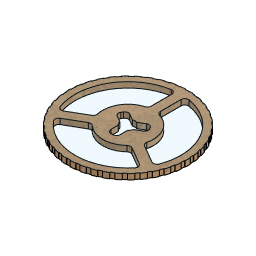
wheel + hub hole v3 (Autodesk Fusion 360 design; units mm, degrees)
Autodesk Fusion 360 part; units mm, degrees
note: some values were not read from the file. Chosen so that the rebuilt part matches the saved one: which bodies a step acts on.
sketch "Sketch1" plane through (0, 0, 0) normal (0, 0, 1) x (1, 0, 0)
  line L0 (-14.6554, 9.616) -> (-15.6554, 7.884)
  arc A0 (14.6554, 9.616) -> (9.1913, 11.0801) centre (11.1913, 7.616) ccw
  line L1 (-1, -17.5) -> (1, -17.5)
  arc A1 (2.3412, 7.1252) -> (-2.3412, 7.1252) centre (0, 0) ccw
  line L2 (15.6554, 7.884) -> (14.6554, 9.616)
  arc A2 (1, -17.5) -> (5, -13.5) centre (1, -13.5) ccw
  arc A3 (-5, -13.5) -> (-1, -17.5) centre (-1, -13.5) ccw
  arc A4 (-15.6554, 7.884) -> (-14.1913, 2.4199) centre (-12.1913, 5.884) ccw
  arc A5 (5, -5.5902) -> (7.3412, -1.535) centre (0, 0) ccw
  arc A6 (14.1913, 2.4199) -> (15.6554, 7.884) centre (12.1913, 5.884) ccw
  line L3 (-14.1913, 2.4199) -> (-7.3412, -1.535)
  arc A7 (-9.1913, 11.0801) -> (-14.6554, 9.616) centre (-11.1913, 7.616) ccw
  line L4 (-5, -5.5902) -> (-5, -13.5)
  line L5 (7.3412, -1.535) -> (14.1913, 2.4199)
  arc A8 (-7.3412, -1.535) -> (-5, -5.5902) centre (0, 0) ccw
  line L6 (-2.3412, 7.1252) -> (-9.1913, 11.0801)
  line L7 (5, -13.5) -> (5, -5.5902)
  line L8 (9.1913, 11.0801) -> (2.3412, 7.1252)
  circle A9 centre (0, 0) radius 65
  dimension "d1" = 130
  constraint concentric A1 A9
  measures "d1" diameter of A9
extrude "Extrude1" add sketch "Sketch1" against normal blind 6 makes body 1
sketch "Sketch2" plane through (0, 0, 0) normal (0, 0, 1) x (-1, 0, 0)
  line L0 (-2.3412, -7.1252) -> (-9.1913, -11.0801)
  arc A0 (-14.6554, -9.616) -> (-9.1913, -11.0801) centre (-11.1913, -7.616) ccw
  line L1 (-14.6554, -9.616) -> (-15.6554, -7.884)
  arc A1 (-14.1913, -2.4199) -> (-15.6554, -7.884) centre (-12.1913, -5.884) ccw
  line L2 (-14.1913, -2.4199) -> (-7.3412, 1.535)
  arc A2 (-5, 5.5902) -> (-7.3412, 1.535) centre (0, 0) ccw
  line L3 (-5, 5.5902) -> (-5, 13.5)
  arc A3 (-1, 17.5) -> (-5, 13.5) centre (-1, 13.5) ccw
  line L4 (-1, 17.5) -> (1, 17.5)
  arc A4 (5, 13.5) -> (1, 17.5) centre (1, 13.5) ccw
  line L5 (5, 13.5) -> (5, 5.5902)
  arc A5 (7.3412, 1.535) -> (5, 5.5902) centre (0, 0) ccw
  line L6 (7.3412, 1.535) -> (14.1913, -2.4199)
  arc A6 (15.6554, -7.884) -> (14.1913, -2.4199) centre (12.1913, -5.884) ccw
  line L7 (15.6554, -7.884) -> (14.6554, -9.616)
  arc A7 (9.1913, -11.0801) -> (14.6554, -9.616) centre (11.1913, -7.616) ccw
  line L8 (9.1913, -11.0801) -> (2.3412, -7.1252)
  arc A8 (-2.3412, -7.1252) -> (2.3412, -7.1252) centre (0, 0) ccw
  circle A9 centre (0, 0) radius 65
  circle A10 centre (0, 0) radius 27.5
  circle A11 centre (0, 0) radius 57.5
  dimension "d4" = 55
  dimension "d5" = 115
  constraint concentric A2 A10
  constraint concentric A2 A11
  measures "d4" diameter of A10
  measures "d5" diameter of A11
extrude "Extrude2" cut sketch "Sketch2" against normal blind 6 contours A11 bodies 1 makes body 2 at (62.0439, -6.0859, 0)
sketch "Sketch3" plane through (0, 0, 0) normal (0, 0, 1) x (-1, 0, 0)
  circle A0 centre (0, 0) radius 27.5
  line L0 (-2.3412, -7.1252) -> (-9.1913, -11.0801)
  arc A1 (-14.6554, -9.616) -> (-9.1913, -11.0801) centre (-11.1913, -7.616) ccw
  line L1 (-14.6554, -9.616) -> (-15.6554, -7.884)
  arc A2 (-14.1913, -2.4199) -> (-15.6554, -7.884) centre (-12.1913, -5.884) ccw
  line L2 (-14.1913, -2.4199) -> (-7.3412, 1.535)
  arc A3 (-5, 5.5902) -> (-7.3412, 1.535) centre (0, 0) ccw
  line L3 (-5, 5.5902) -> (-5, 13.5)
  arc A4 (-1, 17.5) -> (-5, 13.5) centre (-1, 13.5) ccw
  line L4 (-1, 17.5) -> (1, 17.5)
  arc A5 (5, 13.5) -> (1, 17.5) centre (1, 13.5) ccw
  line L5 (5, 13.5) -> (5, 5.5902)
  arc A6 (7.3412, 1.535) -> (5, 5.5902) centre (0, 0) ccw
  line L6 (7.3412, 1.535) -> (14.1913, -2.4199)
  arc A7 (15.6554, -7.884) -> (14.1913, -2.4199) centre (12.1913, -5.884) ccw
  line L7 (15.6554, -7.884) -> (14.6554, -9.616)
  arc A8 (9.1913, -11.0801) -> (14.6554, -9.616) centre (11.1913, -7.616) ccw
  line L8 (9.1913, -11.0801) -> (2.3412, -7.1252)
  arc A9 (-2.3412, -7.1252) -> (2.3412, -7.1252) centre (0, 0) ccw
  line L9 (0, -27.5) -> (0, -58) construction
  line L10 (0, -58) -> (-5, -58) construction
  line L11 (-5, -58) -> (-5, -26) construction
  line L12 (-5, -26) -> (5, -26) construction
  line L13 (5, -26) -> (5, -58) construction
  line L14 (0, -58) -> (5, -58) construction
  line L15 (5, -27.0416) -> (5, -58)
  line L16 (5, -58) -> (-5, -58)
  line L17 (-5, -58) -> (-5, -26)
  line L18 (-5, -26) -> (5, -26)
  line L19 (5, -27.0416) -> (5, -26)
  line L20 (25.0167, 8.6699) -> (20.0167, 17.3301)
  line L21 (20.9187, 17.8509) -> (20.0167, 17.3301)
  line L22 (20.9187, 17.8509) -> (47.7295, 33.3301)
  line L23 (52.7295, 24.6699) -> (25.0167, 8.6699) construction
  line L24 (47.7295, 33.3301) -> (52.7295, 24.6699)
  line L25 (-20.0167, 17.3301) -> (-25.0167, 8.6699)
  line L26 (-25.9187, 9.1907) -> (-25.0167, 8.6699)
  line L27 (-25.9187, 9.1907) -> (-52.7295, 24.6699)
  line L28 (-47.7295, 33.3301) -> (-20.0167, 17.3301) construction
  line L29 (-52.7295, 24.6699) -> (-47.7295, 33.3301)
  line L30 (-20.0167, 17.3301) -> (-47.7295, 33.3301)
  line L31 (25.0167, 8.6699) -> (52.7295, 24.6699)
  dimension "d9" = 360
  constraint coincident A0 L9.start
  constraint vertical L9
  constraint perpendicular L9 L10
  constraint perpendicular L10 L11
  constraint perpendicular L11 L12
  constraint perpendicular L12 L13
  constraint perpendicular L13 L14
  constraint coincident L13 L15.start
  constraint coincident A0 L15.start
  constraint perpendicular L11 L16
  constraint perpendicular L12 L19
extrude "Extrude3" add sketch "Sketch3" against normal blind 6 contours A0 L15 L16 L17 | A0 L22 L24 L31 | A0 L27 L29 L30 bodies 1 2
fillet "Fillet1" radius 4 12 edges at (-20.9187, -17.8509, -3) (-25.9187, -9.1907, -3) (-47.1078, -32.9712, -3) (-52.1078, -24.311, -3) (20.9187, -17.8509, -3) (25.9187, -9.1907, -3) (47.1078, -32.9712, -3) (52.1078, -24.311, -3) (5, 57.2822, -3) (-5, 57.2822, -3) (5, 27.0416, -3) (-5, 27.0416, -3) on bodies 1
sketch "Sketch4" plane through (0, 0, -6) normal (0, 0, -1) x (1, 0, 0)
  arc A0 (9.6729, -56.6806) -> (53.9232, 19.9633) centre (0, 0) ccw
  arc A1 (5, -52.7376) -> (9.6729, -56.6806) centre (9, -52.7376) ccw
  line L0 (5, -52.7376) -> (5, -30.1869)
  arc A2 (7.8571, -26.3537) -> (5, -30.1869) centre (9, -30.1869) ccw
  arc A3 (7.8571, -26.3537) -> (26.7515, 6.3723) centre (0, 0) ccw
  arc A4 (28.6426, 10.7633) -> (26.7515, 6.3723) centre (30.6426, 7.2992) ccw
  line L1 (28.6426, 10.7633) -> (48.1721, 22.0387)
  arc A5 (53.9232, 19.9633) -> (48.1721, 22.0387) centre (50.1721, 18.5746) ccw
  line L2 (43.1721, 30.6989) -> (23.6426, 19.4236)
  arc A6 (18.8944, 19.9813) -> (23.6426, 19.4236) centre (21.6426, 22.8877) ccw
  arc A7 (18.8944, 19.9813) -> (-18.8944, 19.9813) centre (0, 0) ccw
  arc A8 (-23.6426, 19.4236) -> (-18.8944, 19.9813) centre (-21.6426, 22.8877) ccw
  line L3 (-23.6426, 19.4236) -> (-43.1721, 30.6989)
  arc A9 (-44.2503, 36.7173) -> (-43.1721, 30.6989) centre (-41.1721, 34.163) ccw
  arc A10 (44.2503, 36.7173) -> (-44.2503, 36.7173) centre (0, 0) ccw
  arc A11 (43.1721, 30.6989) -> (44.2503, 36.7173) centre (41.1721, 34.163) ccw
  line L4 (-5, -30.1869) -> (-5, -52.7376)
  arc A12 (-9.6729, -56.6806) -> (-5, -52.7376) centre (-9, -52.7376) ccw
  arc A13 (-53.9232, 19.9633) -> (-9.6729, -56.6806) centre (0, 0) ccw
  arc A14 (-48.1721, 22.0387) -> (-53.9232, 19.9633) centre (-50.1721, 18.5746) ccw
  line L5 (-48.1721, 22.0387) -> (-28.6426, 10.7633)
  arc A15 (-26.7515, 6.3723) -> (-28.6426, 10.7633) centre (-30.6426, 7.2992) ccw
  arc A16 (-26.7515, 6.3723) -> (-7.8571, -26.3537) centre (0, 0) ccw
  arc A17 (-5, -30.1869) -> (-7.8571, -26.3537) centre (-9, -30.1869) ccw
  circle A18 centre (0, 0) radius 65
  line L6 (9.1913, -11.0801) -> (2.3412, -7.1252)
  arc A19 (-2.3412, -7.1252) -> (2.3412, -7.1252) centre (0, 0) ccw
  line L7 (-2.3412, -7.1252) -> (-9.1913, -11.0801)
  arc A20 (-14.6554, -9.616) -> (-9.1913, -11.0801) centre (-11.1913, -7.616) ccw
  line L8 (-14.6554, -9.616) -> (-15.6554, -7.884)
  arc A21 (-14.1913, -2.4199) -> (-15.6554, -7.884) centre (-12.1913, -5.884) ccw
  line L9 (-14.1913, -2.4199) -> (-7.3412, 1.535)
  arc A22 (-5, 5.5902) -> (-7.3412, 1.535) centre (0, 0) ccw
  line L10 (-5, 5.5902) -> (-5, 13.5)
  arc A23 (-1, 17.5) -> (-5, 13.5) centre (-1, 13.5) ccw
  line L11 (-1, 17.5) -> (1, 17.5)
  arc A24 (5, 13.5) -> (1, 17.5) centre (1, 13.5) ccw
  line L12 (5, 13.5) -> (5, 5.5902)
  arc A25 (7.3412, 1.535) -> (5, 5.5902) centre (0, 0) ccw
  line L13 (7.3412, 1.535) -> (14.1913, -2.4199)
  arc A26 (15.6554, -7.884) -> (14.1913, -2.4199) centre (12.1913, -5.884) ccw
  line L14 (15.6554, -7.884) -> (14.6554, -9.616)
  arc A27 (9.1913, -11.0801) -> (14.6554, -9.616) centre (11.1913, -7.616) ccw
  line L15 (2, -65.5) -> (-2, -65.5) construction
  line L16 (-2, -65.5) -> (-2, -64.5) construction
  line L17 (-2, -64.5) -> (2, -64.5) construction
  line L18 (2, -64.5) -> (2, -65.5) construction
  line L19 (2, -65.5) -> (-2, -64.5) construction
  line L20 (-2, -65.5) -> (2, -64.5) construction
  line L21 (-2, -64.5) -> (2, -64.5) construction
  line L22 (2, -64.5) -> (2, -65.5) construction
  line L23 (2, -65.5) -> (-2, -65.5) construction
  line L24 (-2, -65.5) -> (-2, -64.5) construction
  line L25 (-2, -64.5) -> (2, -64.5)
  line L26 (2, -64.5) -> (2, -65.5)
  line L27 (2, -65.5) -> (-2, -65.5)
  line L28 (-2, -65.5) -> (-2, -64.5)
  point P0 (0, -65)
  dimension "d14" = 1
  constraint horizontal L15
  constraint perpendicular L15 L16
  constraint parallel L15 L17
  constraint parallel L16 L18
  constraint coincident L19 P0
  constraint coincident L20 P0
  constraint coincident A18 P0
  constraint horizontal L21
  constraint vertical L22
  constraint horizontal L23
  constraint vertical L24
  constraint horizontal L25
  constraint vertical L26
  constraint horizontal L27
  constraint vertical L28
  measures "d14" distance of L15.end L16.end
extrude "Extrude4" cut sketch "Sketch4" against normal blind 6 contours A18 L25 L26 L28 picked at (-0.2223, -64.6655) bodies 1
pattern_circular "C-Pattern1" count 42 over 360 about axis through (0, 0, 1.75) along (0, 0, 1) of "Extrude4"
sketch "Sketch5" plane through (0, 0, 0) normal (0, 0, 1) x (-1, 0, 0)
  line L0 (-11.6608, -63.9455) -> (-11.5909, -63.4815)
  line L1 (-11.5909, -63.4815) -> (-7.6356, -64.0777)
  line L2 (-7.6356, -64.0777) -> (-7.7055, -64.5417)
  arc A0 (-7.7055, -64.5417) -> (-2, -64.9692) centre (0, 0) ccw
  line L3 (-2, -64.9692) -> (-2, -64.5)
  line L4 (-2, -64.5) -> (2, -64.5)
  line L5 (2, -64.5) -> (2, -64.9692)
  arc A1 (2, -64.9692) -> (7.7055, -64.5417) centre (0, 0) ccw
  line L6 (7.7055, -64.5417) -> (7.6356, -64.0777)
  line L7 (7.6356, -64.0777) -> (11.5909, -63.4815)
  line L8 (11.5909, -63.4815) -> (11.6608, -63.9455)
  arc A2 (11.6608, -63.9455) -> (17.2389, -62.6723) centre (0, 0) ccw
  line L9 (17.2389, -62.6723) -> (17.1006, -62.224)
  line L10 (17.1006, -62.224) -> (20.9229, -61.0449)
  line L11 (20.9229, -61.0449) -> (21.0612, -61.4933)
  arc A3 (21.0612, -61.4933) -> (26.3872, -59.403) centre (0, 0) ccw
  line L12 (26.3872, -59.403) -> (26.1836, -58.9803)
  line L13 (26.1836, -58.9803) -> (29.7874, -57.2447)
  line L14 (29.7874, -57.2447) -> (29.991, -57.6675)
  arc A4 (29.991, -57.6675) -> (34.946, -54.8067) centre (0, 0) ccw
  line L15 (34.946, -54.8067) -> (34.6817, -54.419)
  line L16 (34.6817, -54.419) -> (37.9866, -52.1658)
  line L17 (37.9866, -52.1658) -> (38.2509, -52.5535)
  arc A5 (38.2509, -52.5535) -> (42.7242, -48.9862) centre (0, 0) ccw
  line L18 (42.7242, -48.9862) -> (42.405, -48.6422)
  line L19 (42.405, -48.6422) -> (45.3372, -45.9215)
  line L20 (45.3372, -45.9215) -> (45.6564, -46.2655)
  arc A6 (45.6564, -46.2655) -> (49.548, -42.0713) centre (0, 0) ccw
  line L21 (49.548, -42.0713) -> (49.1812, -41.7788)
  line L22 (49.1812, -41.7788) -> (51.6751, -38.6514)
  line L23 (51.6751, -38.6514) -> (52.042, -38.944)
  arc A7 (52.042, -38.944) -> (55.265, -34.2167) centre (0, 0) ccw
  line L24 (55.265, -34.2167) -> (54.8586, -33.9821)
  line L25 (54.8586, -33.9821) -> (56.8586, -30.5179)
  line L26 (56.8586, -30.5179) -> (57.265, -30.7526)
  arc A8 (57.265, -30.7526) -> (59.7475, -25.5977) centre (0, 0) ccw
  line L27 (59.7475, -25.5977) -> (59.3107, -25.4262)
  line L28 (59.3107, -25.4262) -> (60.772, -21.7027)
  line L29 (60.772, -21.7027) -> (61.2088, -21.8742)
  arc A9 (61.2088, -21.8742) -> (62.8953, -16.4069) centre (0, 0) ccw
  line L30 (62.8953, -16.4069) -> (62.4378, -16.3025)
  line L31 (62.4378, -16.3025) -> (63.3279, -12.4027)
  line L32 (63.3279, -12.4027) -> (63.7854, -12.5072)
  arc A10 (63.7854, -12.5072) -> (64.6381, -6.8496) centre (0, 0) ccw
  line L33 (64.6381, -6.8496) -> (64.1702, -6.8145)
  line L34 (64.1702, -6.8145) -> (64.4691, -2.8257)
  line L35 (64.4691, -2.8257) -> (64.937, -2.8607)
  arc A11 (64.937, -2.8607) -> (64.937, 2.8607) centre (0, 0) ccw
  line L36 (64.937, 2.8607) -> (64.4691, 2.8257)
  line L37 (64.4691, 2.8257) -> (64.1702, 6.8145)
  line L38 (64.1702, 6.8145) -> (64.6381, 6.8496)
  arc A12 (64.6381, 6.8496) -> (63.7854, 12.5072) centre (0, 0) ccw
  line L39 (63.7854, 12.5072) -> (63.3279, 12.4027)
  line L40 (63.3279, 12.4027) -> (62.4378, 16.3025)
  line L41 (62.4378, 16.3025) -> (62.8953, 16.4069)
  arc A13 (62.8953, 16.4069) -> (61.2088, 21.8742) centre (0, 0) ccw
  line L42 (61.2088, 21.8742) -> (60.772, 21.7027)
  line L43 (60.772, 21.7027) -> (59.3107, 25.4262)
  line L44 (59.3107, 25.4262) -> (59.7475, 25.5977)
  arc A14 (59.7475, 25.5977) -> (57.265, 30.7526) centre (0, 0) ccw
  line L45 (57.265, 30.7526) -> (56.8586, 30.5179)
  line L46 (56.8586, 30.5179) -> (54.8586, 33.9821)
  line L47 (54.8586, 33.9821) -> (55.265, 34.2167)
  arc A15 (55.265, 34.2167) -> (52.042, 38.944) centre (0, 0) ccw
  line L48 (52.042, 38.944) -> (51.6751, 38.6514)
  line L49 (51.6751, 38.6514) -> (49.1812, 41.7788)
  line L50 (49.1812, 41.7788) -> (49.548, 42.0713)
  arc A16 (49.548, 42.0713) -> (45.6564, 46.2655) centre (0, 0) ccw
  line L51 (45.6564, 46.2655) -> (45.3372, 45.9215)
  line L52 (45.3372, 45.9215) -> (42.405, 48.6422)
  line L53 (42.405, 48.6422) -> (42.7242, 48.9862)
  arc A17 (42.7242, 48.9862) -> (38.2509, 52.5535) centre (0, 0) ccw
  line L54 (38.2509, 52.5535) -> (37.9866, 52.1658)
  line L55 (37.9866, 52.1658) -> (34.6817, 54.419)
  line L56 (34.6817, 54.419) -> (34.946, 54.8067)
  arc A18 (34.946, 54.8067) -> (29.991, 57.6675) centre (0, 0) ccw
  line L57 (29.991, 57.6675) -> (29.7874, 57.2447)
  line L58 (29.7874, 57.2447) -> (26.1836, 58.9803)
  line L59 (26.1836, 58.9803) -> (26.3872, 59.403)
  arc A19 (26.3872, 59.403) -> (21.0612, 61.4933) centre (0, 0) ccw
  line L60 (21.0612, 61.4933) -> (20.9229, 61.0449)
  line L61 (20.9229, 61.0449) -> (17.1006, 62.224)
  line L62 (17.1006, 62.224) -> (17.2389, 62.6723)
  arc A20 (17.2389, 62.6723) -> (11.6608, 63.9455) centre (0, 0) ccw
  line L63 (11.6608, 63.9455) -> (11.5909, 63.4815)
  line L64 (11.5909, 63.4815) -> (7.6356, 64.0777)
  line L65 (7.6356, 64.0777) -> (7.7055, 64.5417)
  arc A21 (7.7055, 64.5417) -> (2, 64.9692) centre (0, 0) ccw
  line L66 (2, 64.9692) -> (2, 64.5)
  line L67 (2, 64.5) -> (-2, 64.5)
  line L68 (-2, 64.5) -> (-2, 64.9692)
  arc A22 (-2, 64.9692) -> (-7.7055, 64.5417) centre (0, 0) ccw
  line L69 (-7.7055, 64.5417) -> (-7.6356, 64.0777)
  line L70 (-7.6356, 64.0777) -> (-11.5909, 63.4815)
  line L71 (-11.5909, 63.4815) -> (-11.6608, 63.9455)
  arc A23 (-11.6608, 63.9455) -> (-17.2389, 62.6723) centre (0, 0) ccw
  line L72 (-17.2389, 62.6723) -> (-17.1006, 62.224)
  line L73 (-17.1006, 62.224) -> (-20.9229, 61.0449)
  line L74 (-20.9229, 61.0449) -> (-21.0612, 61.4933)
  arc A24 (-21.0612, 61.4933) -> (-26.3872, 59.403) centre (0, 0) ccw
  line L75 (-26.3872, 59.403) -> (-26.1836, 58.9803)
  line L76 (-26.1836, 58.9803) -> (-29.7874, 57.2447)
  line L77 (-29.7874, 57.2447) -> (-29.991, 57.6675)
  arc A25 (-29.991, 57.6675) -> (-34.946, 54.8067) centre (0, 0) ccw
  line L78 (-34.946, 54.8067) -> (-34.6817, 54.419)
  line L79 (-34.6817, 54.419) -> (-37.9866, 52.1658)
  line L80 (-37.9866, 52.1658) -> (-38.2509, 52.5535)
  arc A26 (-38.2509, 52.5535) -> (-42.7242, 48.9862) centre (0, 0) ccw
  line L81 (-42.7242, 48.9862) -> (-42.405, 48.6422)
  line L82 (-42.405, 48.6422) -> (-45.3372, 45.9215)
  line L83 (-45.3372, 45.9215) -> (-45.6564, 46.2655)
  arc A27 (-45.6564, 46.2655) -> (-49.548, 42.0713) centre (0, 0) ccw
  line L84 (-49.548, 42.0713) -> (-49.1812, 41.7788)
  line L85 (-49.1812, 41.7788) -> (-51.6751, 38.6514)
  line L86 (-51.6751, 38.6514) -> (-52.042, 38.944)
  arc A28 (-52.042, 38.944) -> (-55.265, 34.2167) centre (0, 0) ccw
  line L87 (-55.265, 34.2167) -> (-54.8586, 33.9821)
  line L88 (-54.8586, 33.9821) -> (-56.8586, 30.5179)
  line L89 (-56.8586, 30.5179) -> (-57.265, 30.7526)
  arc A29 (-57.265, 30.7526) -> (-59.7475, 25.5977) centre (0, 0) ccw
  line L90 (-59.7475, 25.5977) -> (-59.3107, 25.4262)
  line L91 (-59.3107, 25.4262) -> (-60.772, 21.7027)
  line L92 (-60.772, 21.7027) -> (-61.2088, 21.8742)
  arc A30 (-61.2088, 21.8742) -> (-62.8953, 16.4069) centre (0, 0) ccw
  line L93 (-62.8953, 16.4069) -> (-62.4378, 16.3025)
  line L94 (-62.4378, 16.3025) -> (-63.3279, 12.4027)
  line L95 (-63.3279, 12.4027) -> (-63.7854, 12.5072)
  arc A31 (-63.7854, 12.5072) -> (-64.6381, 6.8496) centre (0, 0) ccw
  line L96 (-64.6381, 6.8496) -> (-64.1702, 6.8145)
  line L97 (-64.1702, 6.8145) -> (-64.4691, 2.8257)
  line L98 (-64.4691, 2.8257) -> (-64.937, 2.8607)
  arc A32 (-64.937, 2.8607) -> (-64.937, -2.8607) centre (0, 0) ccw
  line L99 (-64.937, -2.8607) -> (-64.4691, -2.8257)
  line L100 (-64.4691, -2.8257) -> (-64.1702, -6.8145)
  line L101 (-64.1702, -6.8145) -> (-64.6381, -6.8496)
  arc A33 (-64.6381, -6.8496) -> (-63.7854, -12.5072) centre (0, 0) ccw
  line L102 (-63.7854, -12.5072) -> (-63.3279, -12.4027)
  line L103 (-63.3279, -12.4027) -> (-62.4378, -16.3025)
  line L104 (-62.4378, -16.3025) -> (-62.8953, -16.4069)
  arc A34 (-62.8953, -16.4069) -> (-61.2088, -21.8742) centre (0, 0) ccw
  line L105 (-61.2088, -21.8742) -> (-60.772, -21.7027)
  line L106 (-60.772, -21.7027) -> (-59.3107, -25.4262)
  line L107 (-59.3107, -25.4262) -> (-59.7475, -25.5977)
  arc A35 (-59.7475, -25.5977) -> (-57.265, -30.7526) centre (0, 0) ccw
  line L108 (-57.265, -30.7526) -> (-56.8586, -30.5179)
  line L109 (-56.8586, -30.5179) -> (-54.8586, -33.9821)
  line L110 (-54.8586, -33.9821) -> (-55.265, -34.2167)
  arc A36 (-55.265, -34.2167) -> (-52.042, -38.944) centre (0, 0) ccw
  line L111 (-52.042, -38.944) -> (-51.6751, -38.6514)
  line L112 (-51.6751, -38.6514) -> (-49.1812, -41.7788)
  line L113 (-49.1812, -41.7788) -> (-49.548, -42.0713)
  arc A37 (-49.548, -42.0713) -> (-45.6564, -46.2655) centre (0, 0) ccw
  line L114 (-45.6564, -46.2655) -> (-45.3372, -45.9215)
  line L115 (-45.3372, -45.9215) -> (-42.405, -48.6422)
  line L116 (-42.405, -48.6422) -> (-42.7242, -48.9862)
  arc A38 (-42.7242, -48.9862) -> (-38.2509, -52.5535) centre (0, 0) ccw
  line L117 (-38.2509, -52.5535) -> (-37.9866, -52.1658)
  line L118 (-37.9866, -52.1658) -> (-34.6817, -54.419)
  line L119 (-34.6817, -54.419) -> (-34.946, -54.8067)
  arc A39 (-34.946, -54.8067) -> (-29.991, -57.6675) centre (0, 0) ccw
  line L120 (-29.991, -57.6675) -> (-29.7874, -57.2447)
  line L121 (-29.7874, -57.2447) -> (-26.1836, -58.9803)
  line L122 (-26.1836, -58.9803) -> (-26.3872, -59.403)
  arc A40 (-26.3872, -59.403) -> (-21.0612, -61.4933) centre (0, 0) ccw
  line L123 (-21.0612, -61.4933) -> (-20.9229, -61.0449)
  line L124 (-20.9229, -61.0449) -> (-17.1006, -62.224)
  line L125 (-17.1006, -62.224) -> (-17.2389, -62.6723)
  arc A41 (-17.2389, -62.6723) -> (-11.6608, -63.9455) centre (0, 0) ccw
  arc A42 (44.2503, 36.7173) -> (-44.2503, 36.7173) centre (0, 0) ccw
  arc A43 (43.1721, 30.6989) -> (44.2503, 36.7173) centre (41.1721, 34.163) ccw
  line L126 (43.1721, 30.6989) -> (23.6426, 19.4236)
  arc A44 (18.8944, 19.9813) -> (23.6426, 19.4236) centre (21.6426, 22.8877) ccw
  arc A45 (18.8944, 19.9813) -> (-18.8944, 19.9813) centre (0, 0) ccw
  arc A46 (-23.6426, 19.4236) -> (-18.8944, 19.9813) centre (-21.6426, 22.8877) ccw
  line L127 (-23.6426, 19.4236) -> (-43.1721, 30.6989)
  arc A47 (-44.2503, 36.7173) -> (-43.1721, 30.6989) centre (-41.1721, 34.163) ccw
  arc A48 (-26.7515, 6.3723) -> (-7.8571, -26.3537) centre (0, 0) ccw
  arc A49 (-5, -30.1869) -> (-7.8571, -26.3537) centre (-9, -30.1869) ccw
  line L128 (-5, -30.1869) -> (-5, -52.7376)
  arc A50 (-9.6729, -56.6806) -> (-5, -52.7376) centre (-9, -52.7376) ccw
  arc A51 (-53.9232, 19.9633) -> (-9.6729, -56.6806) centre (0, 0) ccw
  arc A52 (-48.1721, 22.0387) -> (-53.9232, 19.9633) centre (-50.1721, 18.5746) ccw
  line L129 (-48.1721, 22.0387) -> (-28.6426, 10.7633)
  arc A53 (-26.7515, 6.3723) -> (-28.6426, 10.7633) centre (-30.6426, 7.2992) ccw
  line L130 (-2.3412, -7.1252) -> (-9.1913, -11.0801)
  arc A54 (-14.6554, -9.616) -> (-9.1913, -11.0801) centre (-11.1913, -7.616) ccw
  line L131 (-14.6554, -9.616) -> (-15.6554, -7.884)
  arc A55 (-14.1913, -2.4199) -> (-15.6554, -7.884) centre (-12.1913, -5.884) ccw
  line L132 (-14.1913, -2.4199) -> (-7.3412, 1.535)
  arc A56 (-5, 5.5902) -> (-7.3412, 1.535) centre (0, 0) ccw
  line L133 (-5, 5.5902) -> (-5, 13.5)
  arc A57 (-1, 17.5) -> (-5, 13.5) centre (-1, 13.5) ccw
  line L134 (-1, 17.5) -> (1, 17.5)
  arc A58 (5, 13.5) -> (1, 17.5) centre (1, 13.5) ccw
  line L135 (5, 13.5) -> (5, 5.5902)
  arc A59 (7.3412, 1.535) -> (5, 5.5902) centre (0, 0) ccw
  line L136 (7.3412, 1.535) -> (14.1913, -2.4199)
  arc A60 (15.6554, -7.884) -> (14.1913, -2.4199) centre (12.1913, -5.884) ccw
  line L137 (15.6554, -7.884) -> (14.6554, -9.616)
  arc A61 (9.1913, -11.0801) -> (14.6554, -9.616) centre (11.1913, -7.616) ccw
  line L138 (9.1913, -11.0801) -> (2.3412, -7.1252)
  arc A62 (-2.3412, -7.1252) -> (2.3412, -7.1252) centre (0, 0) ccw
  arc A63 (7.8571, -26.3537) -> (26.7515, 6.3723) centre (0, 0) ccw
  arc A64 (28.6426, 10.7633) -> (26.7515, 6.3723) centre (30.6426, 7.2992) ccw
  line L139 (28.6426, 10.7633) -> (48.1721, 22.0387)
  arc A65 (53.9232, 19.9633) -> (48.1721, 22.0387) centre (50.1721, 18.5746) ccw
  arc A66 (9.6729, -56.6806) -> (53.9232, 19.9633) centre (0, 0) ccw
  arc A67 (5, -52.7376) -> (9.6729, -56.6806) centre (9, -52.7376) ccw
  line L140 (5, -52.7376) -> (5, -30.1869)
  arc A68 (7.8571, -26.3537) -> (5, -30.1869) centre (9, -30.1869) ccw
